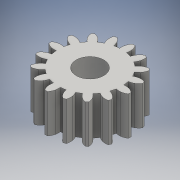
# Autodesk Inventor part: SUPERGEAR12
Saved by Autodesk Inventor 2016 (Build 200138000, 138)
## iProperties
Created: 2018-03-03
Part Number: SUPERGEAR12
Material: Generic
Document SubType Name: Modeling
Designer: Simon
Density: 1 g/cm^3
Appearance: Default
Author: Simon
Autodesk Inventor part; units mm, degrees
ref_plane "YZ Plane" through (0, 0, 0) normal (1, 0, 0) x (0, 1, 0)
ref_plane "XZ Plane" through (0, 0, 0) normal (0, 1, 0) x (-1, 0, 0)
ref_plane "XY Plane" through (0, 0, 0) normal (0, 0, 1) x (1, 0, 0)
sketch "Sketch1" plane through (0, 0, 0) normal (0, 0, 1) x (1, 0, 0)
  circle A0 centre (0, 0) radius 5.7796
  arc A1 (0.9522, 5.7006) -> (1.0134, 6.5519) centre (-3.1591, 6.424) ccw
  arc A2 (1.0134, 6.5519) -> (0.6253, 7.5961) centre (-1.2985, 6.2869) ccw
  arc A3 (-0.3523, 6.6204) -> (-0.3766, 5.7673) centre (3.7864, 6.0754) ccw
  arc A4 (0.1379, 7.6206) -> (-0.3523, 6.6204) centre (1.9217, 6.1262) ccw
  line L0 (0.6253, 7.5961) -> (0.1379, 7.6206)
  arc A5 (0.9522, 5.7006) -> (-0.3766, 5.7673) centre (0, 0) ccw
  arc A6 (-2.7889, 7.0933) -> (-2.859, 5.9817) centre (-0.5689, 6.3953) ccw
  arc A7 (-2.859, 5.9817) -> (-2.555, 5.1842) centre (1.1733, 7.0619) ccw
  line L1 (-2.3292, 7.2572) -> (-2.7889, 7.0933)
  arc A8 (-1.571, 6.441) -> (-2.3292, 7.2572) centre (-3.6056, 5.3114) ccw
  arc A9 (-1.3018, 5.6311) -> (-1.571, 6.441) centre (-5.3769, 4.7261) ccw
  arc A10 (-1.3018, 5.6311) -> (-2.555, 5.1842) centre (0, 0) ccw
  arc A11 (-5.2911, 5.4861) -> (-4.9304, 4.4322) centre (-2.973, 5.6907) ccw
  arc A12 (-4.9304, 4.4322) -> (-4.3444, 3.8118) centre (-1.6185, 6.9733) ccw
  line L2 (-4.9291, 5.8134) -> (-5.2911, 5.4861)
  arc A13 (-3.9163, 5.3495) -> (-4.9291, 5.8134) centre (-5.3637, 3.5273) ccw
  arc A14 (-3.3576, 4.7043) -> (-3.9163, 5.3495) centre (-6.7762, 2.3086) ccw
  arc A15 (-3.3576, 4.7043) -> (-4.3444, 3.8118) centre (0, 0) ccw
  arc A16 (-6.9877, 3.0437) -> (-6.2513, 2.2081) centre (-4.9244, 4.1198) ccw
  arc A17 (-6.2513, 2.2081) -> (-5.4724, 1.8591) centre (-4.1639, 5.8232) ccw
  line L3 (-6.7786, 3.4846) -> (-6.9877, 3.0437)
  arc A18 (-5.6653, 3.4436) -> (-6.7786, 3.4846) centre (-6.3052, 1.2062) ccw
  arc A19 (-4.9023, 3.0613) -> (-5.6653, 3.4436) centre (-7.1439, -0.4602) ccw
  arc A20 (-4.9023, 3.0613) -> (-5.4724, 1.8591) centre (0, 0) ccw
  arc A21 (-7.6206, 0.1379) -> (-6.6204, -0.3523) centre (-6.1262, 1.9217) ccw
  arc A22 (-6.6204, -0.3523) -> (-5.7673, -0.3766) centre (-6.0754, 3.7864) ccw
  line L4 (-7.5961, 0.6253) -> (-7.6206, 0.1379)
  arc A23 (-6.5519, 1.0134) -> (-7.5961, 0.6253) centre (-6.2869, -1.2985) ccw
  arc A24 (-5.7006, 0.9522) -> (-6.5519, 1.0134) centre (-6.424, -3.1591) ccw
  arc A25 (-5.7006, 0.9522) -> (-5.7673, -0.3766) centre (0, 0) ccw
  arc A26 (-7.0933, -2.7889) -> (-5.9817, -2.859) centre (-6.3953, -0.5689) ccw
  arc A27 (-5.9817, -2.859) -> (-5.1842, -2.555) centre (-7.0619, 1.1733) ccw
  line L5 (-7.2572, -2.3292) -> (-7.0933, -2.7889)
  arc A28 (-6.441, -1.571) -> (-7.2572, -2.3292) centre (-5.3114, -3.6056) ccw
  arc A29 (-5.6311, -1.3018) -> (-6.441, -1.571) centre (-4.7261, -5.3769) ccw
  arc A30 (-5.6311, -1.3018) -> (-5.1842, -2.555) centre (0, 0) ccw
  arc A31 (-5.4861, -5.2911) -> (-4.4322, -4.9304) centre (-5.6907, -2.973) ccw
  arc A32 (-4.4322, -4.9304) -> (-3.8118, -4.3444) centre (-6.9733, -1.6185) ccw
  line L6 (-5.8134, -4.9291) -> (-5.4861, -5.2911)
  arc A33 (-5.3495, -3.9163) -> (-5.8134, -4.9291) centre (-3.5273, -5.3637) ccw
  arc A34 (-4.7043, -3.3576) -> (-5.3495, -3.9163) centre (-2.3086, -6.7762) ccw
  arc A35 (-4.7043, -3.3576) -> (-3.8118, -4.3444) centre (0, 0) ccw
  arc A36 (-3.0437, -6.9877) -> (-2.2081, -6.2513) centre (-4.1198, -4.9244) ccw
  arc A37 (-2.2081, -6.2513) -> (-1.8591, -5.4724) centre (-5.8232, -4.1639) ccw
  line L7 (-3.4846, -6.7786) -> (-3.0437, -6.9877)
  arc A38 (-3.4436, -5.6653) -> (-3.4846, -6.7786) centre (-1.2062, -6.3052) ccw
  arc A39 (-3.0613, -4.9023) -> (-3.4436, -5.6653) centre (0.4602, -7.1439) ccw
  arc A40 (-3.0613, -4.9023) -> (-1.8591, -5.4724) centre (0, 0) ccw
  arc A41 (-0.1379, -7.6206) -> (0.3523, -6.6204) centre (-1.9217, -6.1262) ccw
  arc A42 (0.3523, -6.6204) -> (0.3766, -5.7673) centre (-3.7864, -6.0754) ccw
  line L8 (-0.6253, -7.5961) -> (-0.1379, -7.6206)
  arc A43 (-1.0134, -6.5519) -> (-0.6253, -7.5961) centre (1.2985, -6.2869) ccw
  arc A44 (-0.9522, -5.7006) -> (-1.0134, -6.5519) centre (3.1591, -6.424) ccw
  arc A45 (-0.9522, -5.7006) -> (0.3766, -5.7673) centre (0, 0) ccw
  arc A46 (2.7889, -7.0933) -> (2.859, -5.9817) centre (0.5689, -6.3953) ccw
  arc A47 (2.859, -5.9817) -> (2.555, -5.1842) centre (-1.1733, -7.0619) ccw
  line L9 (2.3292, -7.2572) -> (2.7889, -7.0933)
  arc A48 (1.571, -6.441) -> (2.3292, -7.2572) centre (3.6056, -5.3114) ccw
  arc A49 (1.3018, -5.6311) -> (1.571, -6.441) centre (5.3769, -4.7261) ccw
  arc A50 (1.3018, -5.6311) -> (2.555, -5.1842) centre (0, 0) ccw
  arc A51 (5.2911, -5.4861) -> (4.9304, -4.4322) centre (2.973, -5.6907) ccw
  arc A52 (4.9304, -4.4322) -> (4.3444, -3.8118) centre (1.6185, -6.9733) ccw
  line L10 (4.9291, -5.8134) -> (5.2911, -5.4861)
  arc A53 (3.9163, -5.3495) -> (4.9291, -5.8134) centre (5.3637, -3.5273) ccw
  arc A54 (3.3576, -4.7043) -> (3.9163, -5.3495) centre (6.7762, -2.3086) ccw
  arc A55 (3.3576, -4.7043) -> (4.3444, -3.8118) centre (0, 0) ccw
  arc A56 (6.9877, -3.0437) -> (6.2513, -2.2081) centre (4.9244, -4.1198) ccw
  arc A57 (6.2513, -2.2081) -> (5.4724, -1.8591) centre (4.1639, -5.8232) ccw
  line L11 (6.7786, -3.4846) -> (6.9877, -3.0437)
  arc A58 (5.6653, -3.4436) -> (6.7786, -3.4846) centre (6.3052, -1.2062) ccw
  arc A59 (4.9023, -3.0613) -> (5.6653, -3.4436) centre (7.1439, 0.4602) ccw
  arc A60 (4.9023, -3.0613) -> (5.4724, -1.8591) centre (0, 0) ccw
  arc A61 (7.6206, -0.1379) -> (6.6204, 0.3523) centre (6.1262, -1.9217) ccw
  arc A62 (6.6204, 0.3523) -> (5.7673, 0.3766) centre (6.0754, -3.7864) ccw
  line L12 (7.5961, -0.6253) -> (7.6206, -0.1379)
  arc A63 (6.5519, -1.0134) -> (7.5961, -0.6253) centre (6.2869, 1.2985) ccw
  arc A64 (5.7006, -0.9522) -> (6.5519, -1.0134) centre (6.424, 3.1591) ccw
  arc A65 (5.7006, -0.9522) -> (5.7673, 0.3766) centre (0, 0) ccw
  arc A66 (7.0933, 2.7889) -> (5.9817, 2.859) centre (6.3953, 0.5689) ccw
  arc A67 (5.9817, 2.859) -> (5.1842, 2.555) centre (7.0619, -1.1733) ccw
  line L13 (7.2572, 2.3292) -> (7.0933, 2.7889)
  arc A68 (6.441, 1.571) -> (7.2572, 2.3292) centre (5.3114, 3.6056) ccw
  arc A69 (5.6311, 1.3018) -> (6.441, 1.571) centre (4.7261, 5.3769) ccw
  arc A70 (5.6311, 1.3018) -> (5.1842, 2.555) centre (0, 0) ccw
  arc A71 (5.4861, 5.2911) -> (4.4322, 4.9304) centre (5.6907, 2.973) ccw
  arc A72 (4.4322, 4.9304) -> (3.8118, 4.3444) centre (6.9733, 1.6185) ccw
  line L14 (5.8134, 4.9291) -> (5.4861, 5.2911)
  arc A73 (5.3495, 3.9163) -> (5.8134, 4.9291) centre (3.5273, 5.3637) ccw
  arc A74 (4.7043, 3.3576) -> (5.3495, 3.9163) centre (2.3086, 6.7762) ccw
  arc A75 (4.7043, 3.3576) -> (3.8118, 4.3444) centre (0, 0) ccw
  arc A76 (3.0437, 6.9877) -> (2.2081, 6.2513) centre (4.1198, 4.9244) ccw
  arc A77 (2.2081, 6.2513) -> (1.8591, 5.4724) centre (5.8232, 4.1639) ccw
  line L15 (3.4846, 6.7786) -> (3.0437, 6.9877)
  arc A78 (3.4436, 5.6653) -> (3.4846, 6.7786) centre (1.2062, 6.3052) ccw
  arc A79 (3.0613, 4.9023) -> (3.4436, 5.6653) centre (-0.4602, 7.1439) ccw
  arc A80 (3.0613, 4.9023) -> (1.8591, 5.4724) centre (0, 0) ccw
  dimension "d22" = 11.5592
  dimension "d18" = 360
  constraints: 160 point on circle, 80 centre point, 32 end point, 277 other
extrude "Extrusion1" add sketch "Sketch1" along normal blind 7
sketch "Sketch2" plane through (0, 0, 7) normal (0, 0, 1) x (1, 0, 0)
  circle A0 centre (0, 0) radius 2.5
  dimension "d23" = 5
  constraints: 1 centre point, 1 coincident
  measures "d23" diameter of A0
extrude "Extrusion2" cut sketch "Sketch2" against normal blind 10
body "Solid1"
